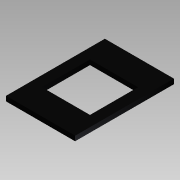
# Autodesk Inventor part: peltier felt
Saved by Autodesk Inventor 2015 (Build 190159000, 159)
## iProperties
Created: 2015-05-21
Part Number: peltier felt
Material: Acetal Resin, Black
Document SubType Name: Modeling
Designer: Joe Sheldon
Density: 1.425 g/cm^3
Appearance: Smooth - Black
Author: Joe Sheldon
Autodesk Inventor part; units mm, degrees
ref_plane "YZ Plane" through (0, 0, 0) normal (1, 0, 0) x (0, 1, 0)
ref_plane "XZ Plane" through (0, 0, 0) normal (0, 1, 0) x (-1, 0, 0)
ref_plane "XY Plane" through (0, 0, 0) normal (0, 0, 1) x (1, 0, 0)
sketch "Sketch1" plane through (0, 0, 0) normal (0, 1, 0) x (-1, 0, 0)
  line L0 (38.1, 0) -> (38.1, -38.1)
  line L1 (0, -38.1) -> (0, 0)
  line L2 (0, 0) -> (0, 11.811)
  line L3 (0, 11.811) -> (38.1, 11.811)
  line L4 (38.1, 11.811) -> (38.1, 0)
  line L5 (0, -38.1) -> (0, -49.911)
  line L6 (0, -49.911) -> (38.1, -49.911)
  line L7 (38.1, -49.911) -> (38.1, -38.1)
  line L8 (-8.382, -38.1) -> (-8.382, -58.293)
  line L9 (-8.382, -58.293) -> (46.482, -58.293)
  line L10 (46.482, -58.293) -> (46.482, -38.1)
  line L11 (46.482, -38.1) -> (46.482, 0)
  line L12 (46.482, 0) -> (46.482, 20.193)
  line L13 (46.482, 20.193) -> (-8.382, 20.193)
  line L14 (-8.382, 20.193) -> (-8.382, 0)
  line L15 (-8.382, 0) -> (-8.382, -38.1)
  dimension "d0" = 38.1
  dimension "d1" = 38.1
  dimension "d2" = 11.811
  dimension "d3" = 11.811
  dimension "d4" = 8.382
  constraints: 32 end point, 5 parallel, 2 point on line, 1 vertical, 6 other
  measures "d0" distance of L0.end L1.start
  measures "d1" distance of L0.start L0.end
  measures "d2" distance of L2.start L2.end
  measures "d3" distance of L5.end L5.start
  measures "d4" distance between parallel lines of L0 L11
extrude "Extrusion1" add sketch "Sketch1" along normal blind 3.81 contours L0 L7 L6 L5 L1 L2 L3 L4 | L15 L14 L13 L12 L11 L10 L9 L8
sketch "Sketch2" plane through (0, 3.81, 0) normal (0, 1, 0) x (1, 0, 0)
  line L0 (0, 0) -> (-38.1, 0)
  line L1 (-38.1, 0) -> (-38.1, 38.1)
  line L2 (-38.1, 38.1) -> (0, 38.1)
  line L3 (0, 38.1) -> (0, 0)
  dimension "d7" = 38.1
  dimension "d8" = 38.1
  constraints: 8 end point, 2 parallel, 1 horizontal, 1 perpendicular
  measures "d7" distance of L1.end L2.end
  measures "d8" distance of L0.end L1.end
extrude "Extrusion2" cut sketch "Sketch2" against normal blind 13.6525
body "Solid1"
